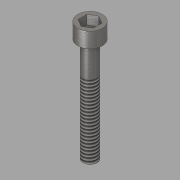
# Autodesk Inventor part: Tube Rack bolt
Saved by Autodesk Inventor 2017 (Build 210142000, 142)
## iProperties
Created: 2017-01-17
Part Number: Tube Rack bolt
Material: Steel, Galvanized
Document SubType Name: Modeling
Designer: qupec
Density: 7.85 g/cm^3
Appearance: Galvanized
Author: qupec
Autodesk Inventor part; units mm, degrees
ref_plane "YZ Plane" through (0, 0, 0) normal (1, 0, 0) x (0, 1, 0)
ref_plane "XZ Plane" through (0, 0, 0) normal (0, 1, 0) x (-1, 0, 0)
ref_plane "XY Plane" through (0, 0, 0) normal (0, 0, 1) x (1, 0, 0)
sketch "Sketch1" plane through (0, 0, 0) normal (0, 1, 0) x (-1, 0, 0)
  circle A0 centre (0, 0) radius 1.4605
  dimension "d0" = 2.921
  constraints: 1 centre point, 1 coincident
  measures "d0" diameter of A0
extrude "Extrusion1" add sketch "Sketch1" along normal blind 21.59
sketch "Sketch2" plane through (0, 21.59, 0) normal (0, 1, 0) x (1, 0, 0)
  circle A0 centre (0, 0) radius 2.54
  dimension "d3" = 5.08
  constraints: 1 centre point, 1 coincident
  measures "d3" diameter of A0
extrude "Extrusion2" add sketch "Sketch2" along normal blind 3.175
sketch "Sketch3" plane through (0, 24.765, 0) normal (0, 1, 0) x (1, 0, 0)
  line L0 (0, 1.8331) -> (1.5875, 0.9165)
  line L1 (1.5875, 0.9165) -> (1.5875, -0.9165)
  line L2 (1.5875, -0.9165) -> (0, -1.8331)
  line L3 (0, -1.8331) -> (-1.5875, -0.9165)
  line L4 (-1.5875, -0.9165) -> (-1.5875, 0.9165)
  line L5 (-1.5875, 0.9165) -> (0, 1.8331)
  point P0 (0, 0)
  point P1 (0, 0)
  dimension "d6" = 3.175
  constraints: 12 end point, 1 coincident, 13 other
  measures "d6" distance between parallel lines of L1 L4
extrude "Extrusion3" cut sketch "Sketch3" against normal blind 1.905
thread "Thread1" size "5-40 UNC" class "2A" standard "ANSI Unified Screw Threads" length 34.29 offset 6.35
body "Solid1"
